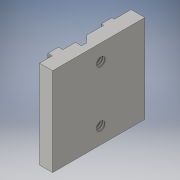
# Autodesk Inventor part: 80-20 extrusion rail
Saved by Autodesk Inventor 2016 SP2 (Build 200236200, 236)
## iProperties
Created: 2018-01-11
Part Number: 80-20 extrusion rail
Material: Generic
Document SubType Name: Modeling
Designer: CAD
Density: 1 g/cm^3
Appearance: Default
Author: CAD
Autodesk Inventor part; units mm, degrees
ref_plane "YZ Plane" through (0, 0, 0) normal (1, 0, 0) x (0, 1, 0)
ref_plane "XZ Plane" through (0, 0, 0) normal (0, 1, 0) x (-1, 0, 0)
ref_plane "XY Plane" through (0, 0, 0) normal (0, 0, 1) x (1, 0, 0)
sketch "Sketch1" plane through (0, 0, 0) normal (0, 1, 0) x (-1, 0, 0)
  line L0 (0, 0) -> (0, -52.6034)
  line L1 (0, -52.6034) -> (7.874, -52.6034)
  line L2 (0, 0) -> (7.493, 0)
  line L3 (7.493, 0) -> (7.493, -7.239)
  line L4 (7.493, -7.239) -> (9.9568, -7.239)
  line L5 (9.9568, -7.239) -> (9.9568, -13.335)
  line L6 (9.9568, -13.335) -> (7.493, -13.335)
  line L7 (7.493, -13.335) -> (7.493, -20.574)
  line L8 (7.493, -20.574) -> (4.064, -20.574)
  line L9 (4.064, -20.574) -> (4.064, -23.368)
  line L10 (7.874, -27.4574) -> (4.064, -23.368)
  line L11 (7.874, -43.0784) -> (9.271, -43.0784)
  line L12 (9.271, -43.0784) -> (9.271, -36.9824)
  line L13 (9.271, -36.9824) -> (7.874, -36.9824)
  line L14 (7.874, -52.6034) -> (7.874, -43.0784)
  line L15 (7.874, -36.9824) -> (7.874, -27.4574)
  dimension "d2" = 52.6034
  dimension "d3" = 7.874
  dimension "d4" = 25.146
  dimension "d5" = 7.493
  dimension "d7" = 2.4638
  dimension "d8" = 6.096
  dimension "d10" = 3.429
  dimension "d11" = 2.794
  dimension "d12" = 20.574
  dimension "d13" = 7.239
  dimension "d14" = 1.397
  dimension "d15" = 6.096
  dimension "d17" = 9.525
  constraints: 32 end point, 13 perpendicular, 2 point on line, 2 vertical, 1 horizontal
  measures "d2" distance of L0.start L0.end
  measures "d3" distance of L0.end L1.end
  measures "d4" distance of L1.end L10.start
  measures "d5" distance of L0.start L2.end
  measures "d7" distance of L3.end L4.end
  measures "d8" distance of L4.end L5.end
  measures "d10" distance of L7.end L8.end
  measures "d11" distance of L8.end L9.end
  measures "d12" distance between parallel lines of L2 L8
  measures "d13" distance between parallel lines of L6 L8
  measures "d14" distance of L11.start L11.end
  measures "d15" distance of L11.end L12.end
  measures "d17" distance between parallel lines of L11 L1
extrude "Extrusion1" add sketch "Sketch1" along normal blind 50.292
sketch "Sketch2" plane through (-7.874, 0, -36.9824) normal (-1, 0, 0) x (0, 0, 1)
  line L0 (9.525, 0) -> (9.525, 50.292) projected
  line L1 (9.525, 0) -> (13.6144, 0) projected
  line L2 (9.525, 50.292) -> (13.6144, 50.292) projected
  point P0 (36.9824, 0)
  point P1 (9.6228, 9.271)
  point P2 (9.525, 41.021)
  dimension "d20" = 31.75
  dimension "d21" = 9.271
  dimension "d22" = 9.271
  constraints: 1 point on line
  measures "d20" vertical distance of point (9.623, 9.271) point (9.525, 41.021)
  measures "d21" distance from line of L1 point (9.623, 9.271)
  measures "d22" distance from line of point (9.525, 41.021) L2
hole "Hole1" at (-7.874, 9.271, -27.3596) at (-7.874, 41.021, -27.4574) direction (1, 0, 0) diameter 4.9784 depth 19.05 tip angle 118 thread size "1/4-20 UNC" class "2B" standard "ANSI Unified Screw Threads"
body "Solid1"
